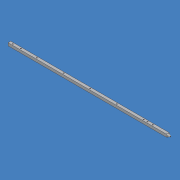
# Autodesk Inventor part: Long rod
Saved by Autodesk Inventor 2011 (Build 150239000, 239)
## iProperties
Created: 2005-07-04
Part Number: Long rod
Document SubType Name: Modeling
Designer: jony
Density: 1 g/cm^3
Author: jony
Autodesk Inventor part; units mm, degrees
ref_plane "YZ Plane" through (0, 0, 0) normal (1, 0, 0) x (0, 1, 0)
ref_plane "XZ Plane" through (0, 0, 0) normal (0, 1, 0) x (-1, 0, 0)
sketch "Sketch1" plane through (0, 0, 0) normal (0, 0, 1) x (1, 0, 0)
  line L0 (-374.9457, 6.7465) -> (391.8168, 6.7465)
  line L1 (391.8168, 6.7465) -> (391.8168, -5.9535)
  line L2 (391.8168, -5.9535) -> (-374.9457, -5.9535)
  line L3 (-374.9457, -5.9535) -> (-374.9457, 6.7465)
  dimension "d0" = 766.7625
  dimension "d1" = 12.7
  constraints: 8 end point, 2 parallel, 1 horizontal, 1 perpendicular
  measures "d0" distance of L0.start L0.end
  measures "d1" distance of L2.end L0.start
extrude "Extrusion1" add sketch "Sketch1" along normal blind 12.7
hole "Hole3" at (-358.4357, 0.3965, 12.7) direction (0, 0, -1) diameter 5 end through all
hole "Hole4" at (-320.3357, 0.3965, 12.7) direction (0, 0, -1) diameter 5 end through all
hole "Hole5" at (-244.2881, 0.3965, 12.7) direction (0, 0, -1) diameter 5 end through all
hole "Hole6" at (-117.2881, 0.3965, 12.7) direction (0, 0, -1) diameter 5 end through all
hole "Hole7" at (9.7119, 0.3965, 12.7) direction (0, 0, -1) diameter 5 end through all
hole "Hole8" at (136.7119, 0.3965, 12.7) direction (0, 0, -1) diameter 5 end through all
hole "Hole9" at (263.7119, 0.3965, 12.7) direction (0, 0, -1) diameter 5 end through all
hole "Hole10" at (281.7967, 0.3965, 12.7) direction (0, 0, -1) diameter 5 end through all
hole "Hole11" at (307.1967, 0.3965, 12.7) direction (0, 0, -1) diameter 5 end through all
hole "Hole12" at (391.8168, 0.3965, 6.35) direction (-1, 0, 0) diameter 3 depth 8 tip angle 118
ref_plane "Work Plane1" through (387.8168, 0.3965, 6.35) normal (0, 0, 1) x (1, 0, 0)
sketch "Sketch4" plane through (387.8168, 0.3965, 6.35) normal (0, 0, 1) x (1, 0, 0)
  line L0 (4, 6.35) -> (4, -6.35) projected
  line L1 (4, 0) -> (-4.9613, 0)
  line L2 (-839.4388, 0) -> (234.0288, 0) projected
  line L3 (4, 2.0193) -> (4, 6.35)
  line L4 (-5.6322, 6.35) -> (4, 2.0193)
  line L5 (-5.6322, 9.0208) -> (4, 9.0208)
  line L6 (4, 9.0208) -> (4, 6.0715)
  line L7 (-5.6322, 6.35) -> (-11.5724, 9.0208)
  line L8 (-5.9043, 9.0208) -> (-11.5724, 9.0208)
  line L9 (-5.6322, 9.0208) -> (-5.9043, 9.0208)
  constraints: 16 end point, 2 collinear, 2 perpendicular, 2 point on line, 1 midpoint
revolve "Revolution2" cut sketch "Sketch4" angle 360 about axis through (391.8168, 0.3965, 6.35) along (-1, 0, 0)
body "Solid1"
